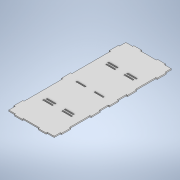
# Autodesk Inventor part: in_separator
Saved by Autodesk Inventor 2020 (Build 240168000, 168)
## iProperties
Created: 2020-02-24
Part Number: in_separator
Material: Generic
Document SubType Name: Modeling
Designer: udvarhelyi
Density: 1 g/cm^3
Appearance: Default
Author: udvarhelyi
Autodesk Inventor part; units mm, degrees
ref_plane "YZ Plane" through (0, 0, 0) normal (1, 0, 0) x (0, 1, 0)
ref_plane "XZ Plane" through (0, 0, 0) normal (0, 1, 0) x (-1, 0, 0)
ref_plane "XY Plane" through (0, 0, 0) normal (0, 0, 1) x (1, 0, 0)
sketch "Sketch1" plane through (0, 0, 0) normal (0, 1, 0) x (-1, 0, 0)
  line L0 (20, 147) -> (20, 150)
  line L1 (20, 150) -> (40, 150)
  line L2 (40, 150) -> (40, 147)
  line L3 (-20, 147) -> (-20, 150)
  line L4 (-20, 150) -> (-40, 150)
  line L5 (-40, 150) -> (-40, 147)
  line L6 (-40, 147) -> (-57, 147)
  line L7 (57, 147) -> (40, 147)
  line L8 (20, 147) -> (-20, 147)
  line L9 (20, -147) -> (20, -150)
  line L10 (20, -150) -> (40, -150)
  line L11 (40, -150) -> (40, -147)
  line L12 (-40, -147) -> (-40, -150)
  line L13 (-40, -150) -> (-20, -150)
  line L14 (-20, -150) -> (-20, -147)
  line L15 (40, -147) -> (57, -147)
  line L16 (-57, -147) -> (-40, -147)
  line L17 (-20, -147) -> (20, -147)
  line L18 (-57, 131.4286) -> (-60, 131.4286)
  line L19 (-60, 131.4286) -> (-60, 108.5714)
  line L20 (-60, 108.5714) -> (-57, 108.5714)
  line L21 (-57, 11.4286) -> (-60, 11.4286)
  line L22 (-60, 11.4286) -> (-60, -11.4286)
  line L23 (-60, -11.4286) -> (-57, -11.4286)
  line L24 (-57, -108.5714) -> (-60, -108.5714)
  line L25 (-60, -108.5714) -> (-60, -131.4286)
  line L26 (-60, -131.4286) -> (-57, -131.4286)
  line L27 (-57, 147) -> (-57, 131.4286)
  line L28 (-57, -131.4286) -> (-57, -147)
  line L29 (57, 131.4286) -> (60, 131.4286)
  line L30 (60, 131.4286) -> (60, 108.5714)
  line L31 (60, 108.5714) -> (57, 108.5714)
  line L32 (57, 11.4286) -> (60, 11.4286)
  line L33 (60, 11.4286) -> (60, -11.4286)
  line L34 (60, -11.4286) -> (57, -11.4286)
  line L35 (57, -108.5714) -> (60, -108.5714)
  line L36 (60, -108.5714) -> (60, -131.4286)
  line L37 (60, -131.4286) -> (57, -131.4286)
  line L38 (57, 131.4286) -> (57, 147)
  line L39 (57, 11.4286) -> (57, 108.5714)
  line L40 (57, -147) -> (57, -131.4286)
  line L41 (57, -108.5714) -> (57, -11.4286)
  line L42 (-57, 57.1429) -> (-60, 57.1429)
  line L43 (-60, 57.1429) -> (-60, 34.2857)
  line L44 (-60, 34.2857) -> (-57, 34.2857)
  line L45 (-57, -34.2857) -> (-60, -34.2857)
  line L46 (-60, -34.2857) -> (-60, -57.1429)
  line L47 (-60, -57.1429) -> (-57, -57.1429)
  line L48 (-57, 108.5714) -> (-57, 57.1429)
  line L49 (-57, 34.2857) -> (-57, 11.4286)
  line L50 (-57, -11.4286) -> (-57, -34.2857)
  line L51 (-57, -57.1429) -> (-57, -108.5714)
  line L52 (-36, 80) -> (-12, 80)
  line L53 (-12, 80) -> (-12, 83)
  line L54 (-12, 83) -> (-36, 83)
  line L55 (-36, 83) -> (-36, 80)
  line L56 (-36, -80) -> (-12, -80)
  line L57 (-12, -80) -> (-12, -83)
  line L58 (-12, -83) -> (-36, -83)
  line L59 (-36, -83) -> (-36, -80)
  line L60 (12, 83) -> (36, 83)
  line L61 (36, 83) -> (36, 80)
  line L62 (36, 80) -> (12, 80)
  line L63 (12, 80) -> (12, 83)
  line L64 (12, -80) -> (36, -80)
  line L65 (36, -80) -> (36, -83)
  line L66 (36, -83) -> (12, -83)
  line L67 (12, -83) -> (12, -80)
  point P0 (0, 0)
  point P1 (-60, 120)
  point P2 (-60, -120)
  dimension "d1" = 294
  dimension "d5" = 20
  dimension "d7" = 20
  dimension "d9" = 3
  dimension "d10" = 147
  dimension "d11" = 3
  dimension "d12" = 57
  dimension "d13" = 3
  dimension "d14" = 17
  dimension "d15" = 3
  dimension "d16" = 17
  dimension "d17" = 22.8571
  dimension "d18" = 11.4286
  dimension "d20" = 120
  dimension "d21" = 17
  dimension "d24" = 114
  dimension "d25" = 22.8571
  dimension "d26" = 24
  dimension "d27" = 3
  dimension "d28" = 3
  dimension "d29" = 22.8571
  dimension "d30" = 24
  dimension "d31" = 24
  dimension "d32" = 22.8571
  dimension "d33" = 120
  constraints: 136 end point, 55 parallel, 30 perpendicular, 25 collinear, 15 horizontal, 13 equal length, 12 point on line, 2 midpoint
  measures "d1" distance of L15.end L7.start
  measures "d5" distance of L0.end L1.end
  measures "d7" distance of L3.end L4.end
  measures "d9" distance of L1.end L2.end
  measures "d10" distance from line of point (0, 0) L17
  measures "d11" distance of L10.end L11.end
  measures "d12" distance from line of point (0, 0) L27
  measures "d13" distance of L18.start L18.end
  measures "d14" distance from line of L38 L1.end
  measures "d15" distance of L29.start L29.end
  measures "d16" distance between parallel lines of L5 L27
  measures "d17" distance of L21.end L22.end
  measures "d18" vertical distance of L21.end point (0, 0)
  measures "d20" vertical distance of point (0, 0) point (-60, 120)
  measures "d21" distance between parallel lines of L28 L12
  measures "d24" distance between parallel lines of L28 L40
  measures "d25" distance between parallel lines of L44 L21
  measures "d26" distance of L53.end L54.end
  measures "d27" distance of L54.end L52.start
  measures "d28" distance of L58.end L56.start
  measures "d29" distance between parallel lines of L52 L42
  measures "d30" distance between parallel lines of L43 L55
  measures "d31" distance between parallel lines of L53 L63
  measures "d32" distance between parallel lines of L47 L56
  measures "d33" vertical distance of point (-60, -120) point (0, 0)
extrude "Extrusion1" add sketch "Sketch1" along normal blind 3
sketch "Sketch2" plane through (0, 3, 0) normal (0, 1, 0) x (1, 0, 0)
  line L0 (34.2, 76.5) -> (11.4, 76.5)
  line L1 (11.4, 76.5) -> (11.4, 73.5)
  line L2 (11.4, 73.5) -> (34.2, 73.5)
  line L3 (34.2, 73.5) -> (34.2, 76.5)
  line L4 (-11.4, 76.5) -> (-34.2, 76.5)
  line L5 (-34.2, 76.5) -> (-34.2, 73.5)
  line L6 (-34.2, 73.5) -> (-11.4, 73.5)
  line L7 (-11.4, 73.5) -> (-11.4, 76.5)
  line L8 (34.2, 73.5) -> (57, 73.5) construction
  line L9 (11.4, 73.5) -> (-11.4, 73.5) construction
  line L10 (-34.2, 73.5) -> (-57, 73.5) construction
  line L11 (-57, 108.5714) -> (-57, 11.4286) projected
  line L12 (57, 57.1429) -> (57, 108.5714) projected
  point P0 (0, 0)
  dimension "d34" = 22.8
  dimension "d35" = 22.8
  dimension "d36" = 3
  dimension "d37" = 73.5
  constraints: 22 end point, 5 point on line, 4 horizontal, 4 parallel, 3 collinear, 2 perpendicular
  measures "d34" distance of L1.end L2.end
  measures "d35" distance of L2.end L8.end
  measures "d36" distance of L2.end L0.start
  measures "d37" distance from line of point (0, 0) L2
extrude "Extrusion2" cut sketch "Sketch2" against normal through all
pattern_linear "Rectangular Pattern1" count 3 spacing 75 along (0, 0, 1) of "Extrusion2"
equation "\"d1\" = wt - 2 * tt"
equation "\"d9\" = tt"
equation "\"d10\" = 0.5 * wt - tt"
equation "\"d11\" = tt"
equation "\"d12\" = 0.5 * ht - tt"
equation "\"d13\" = tt"
equation "\"d15\" = tt"
equation "\"d17\" = 0.142857 * shelfW + 2 * tol"
equation "\"d18\" = 0.0714286 * shelfW + tol"
equation "\"d20\" = 0.4 * wt"
equation "\"d24\" = ht - 2 * tt"
equation "\"d25\" = 0.142857 * shelfW - 2 * tol"
equation "\"d26\" = 0.2 * ht + 2 * tol"
equation "\"d27\" = tt"
equation "\"d28\" = tt"
equation "\"d29\" = 0.142857 * shelfW - tol"
equation "\"d30\" = 0.2 * ht - tol"
equation "\"d31\" = 0.2 * ht - 2 * tol"
equation "\"d32\" = 0.142857 * shelfW - tol"
equation "\"d33\" = 0.4 * wt"
equation "\"d22\" = tt"
equation "\"d34\" = -0.4 * tt + 0.2 * ht + 2 * tol"
equation "\"d36\" = tt"
equation "\"d37\" = 0.25 * wt - 0.5 * tt"
equation "\"d42\" = 0.25 * wt"
equation "\"d0\" = 0.5 * wt - tt"
equation "\"tt\" = 3"
equation "\"tol\" = 0"
equation "\"tiroir\" = 1"
equation "\"nHoles\" = 4"
equation "\"shelfH\" = 35"
equation "\"d3\" = 0.5 * ht - tt"
equation "\"wt\" = 300"
equation "\"shelfW\" = 160"
equation "\"ht\" = 120"
body "Solid1"
